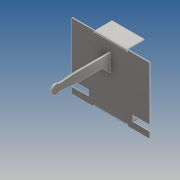
# Autodesk Inventor part: Porta actuador
Saved by Autodesk Inventor 2016 (Build 200138000, 138)
## iProperties
Created: 2016-05-25
Part Number: Porta actuador
Material: Stainless Steel
Document SubType Name: Sheet Metal
Designer: Familia
Density: 8 g/cm^3
Sheet Metal Rule: Default_mm
Appearance: Semi-Polished
Author: Familia
Autodesk Inventor part; units mm, degrees
note: some values were not read from the file. Chosen so that the rebuilt part matches the saved one: relief shape of "Plate2"; relief shape of "Plate3".
ref_plane "YZ Plane" through (0, 0, 0) normal (1, 0, 0) x (0, 1, 0)
ref_plane "XZ Plane" through (0, 0, 0) normal (0, 1, 0) x (-1, 0, 0)
ref_plane "XY Plane" through (0, 0, 0) normal (0, 0, 1) x (1, 0, 0)
sketch "Sketch1" plane through (0, 0, 0) normal (0, 1, 0) x (-1, 0, 0)
  line L0 (26.5, -22.5) -> (-26.5, -22.5)
  line L1 (-26.5, -22.5) -> (-26.5, 22.5)
  line L2 (-26.5, 22.5) -> (26.5, 22.5)
  line L3 (26.5, 22.5) -> (26.5, -22.5)
  line L4 (26.5, -22.5) -> (-26.5, 22.5) construction
  line L5 (-26.5, -22.5) -> (26.5, 22.5) construction
  line L6 (-23.1815, -2.0327) -> (-17.2605, -2.0327)
  line L7 (-17.2605, -2.0327) -> (-17.2605, -20.329)
  line L8 (-17.2605, -20.329) -> (-23.1815, -20.329)
  line L9 (-23.1815, -20.329) -> (-23.1815, -2.0327)
  line L10 (15.4694, -2.0327) -> (21.0827, -2.0327)
  line L11 (21.0827, -2.0327) -> (21.0827, -20.329)
  line L12 (21.0827, -20.329) -> (15.4694, -20.329)
  line L13 (15.4694, -20.329) -> (15.4694, -2.0327)
  line L14 (1, 11) -> (0, 11)
  line L15 (0, 11) -> (0, 3)
  line L16 (0, 3) -> (1, 3)
  line L17 (1, 3) -> (1, 11)
  point P0 (0, 0)
  point P1 (0, 0)
  dimension "d0" = 53
  dimension "d1" = 45
  dimension "d43" = 8
  dimension "d44" = 1
  dimension "d45" = 3
  measures "d0" distance of L1.end L2.end
  measures "d1" distance of L2.end L0.start
  measures "d43" distance of L16.end L14.start
  measures "d44" distance of L14.start L14.end
  measures "d45" distance of point (0, 0) L15.end
extrude "Plate1" add sketch "Sketch1" along normal blind 0.5 contours L0 L1 L2 L3 | L6 L7 L8 L9 | L10 L11 L12 L13 | L17 L16 L15 L14
sketch "Sketch2" plane through (26.5, 0, 22) normal (0, 0, 1) x (1, 0, 0)
  line L0 (-37.5, 0) -> (-15.5, 0)
  line L1 (-15.5, 0) -> (-15.5, 12)
  line L2 (-15.5, 12) -> (-37.5, 12)
  line L3 (-37.5, 12) -> (-37.5, 0)
  constraints: 8 end point
edge flange "Flange1" height 12 angle 90 thickness 0.5 bend radius 0.5 thickness toward (0, 0, 1) relief straight relief width 0.5 relief depth 0.25 edges at (0, 0.5, 22.5) wall of the first edge with corners at (-11, 0, 22) (11, 0, 22) (11, 12, 22) (-11, 12, 22)
bend "Bend1"
corner "Corner1"
sketch "Sketch3" plane through (26.5, 0, -22) normal (0, 0, -1) x (-1, 0, 0)
  line L0 (37.5, 0) -> (15.5, 0)
  line L1 (15.5, 0) -> (15.5, -12)
  line L2 (15.5, -12) -> (37.5, -12)
  line L3 (37.5, -12) -> (37.5, 0)
  constraints: 8 end point
edge flange "Flange2" height 12 angle 90 thickness 0.5 bend radius 0.5 thickness toward (0, 0, -1) relief straight relief width 0.5 relief depth 0.25 edges at (0, 0, -22.5) wall of the first edge with corners at (-11, 0, -22) (11, 0, -22) (11, 12, -22) (-11, 12, -22)
bend "Bend2"
corner "Corner2"
sketch "Sketch4" plane through (0, 0, 0) normal (0, -1, 0) x (1, 0, 0)
  line L0 (-32.114, -14.2) -> (-15, -14.2)
  line L1 (-15, -14.2) -> (-15, -18.2)
  line L2 (-15, -18.2) -> (-32.114, -18.2)
  line L3 (-32.114, -18.2) -> (-32.114, -14.2)
  line L4 (15, -14.2) -> (31.1601, -14.2)
  line L5 (31.1601, -14.2) -> (31.1601, -18.2)
  line L6 (31.1601, -18.2) -> (15, -18.2)
  line L7 (15, -18.2) -> (15, -14.2)
  line L8 (26.5, -22.5) -> (26.5, 22.5) projected
  line L9 (-26.5, 22.5) -> (-26.5, -22.5) projected
  line L10 (-15, -16.2) -> (0, -16.2) construction
  line L11 (0, -16.2) -> (15, -16.2) construction
  line L12 (0, 0) -> (0, -16.2) construction
  dimension "d25" = 4.3
  dimension "d26" = 4.3
  dimension "d27" = 30
  dimension "d29" = 4
  constraints: 22 end point, 4 parallel, 3 horizontal, 2 midpoint, 2 perpendicular, 1 collinear, 1 point on line, 1 vertical
  measures "d25" vertical distance of L2.end L9.end
  measures "d26" distance from line of L6 L8.start
  measures "d27" distance between parallel lines of L7 L1
  measures "d29" distance of L4.end L5.end
extrude "Cut1" cut sketch "Sketch4" against normal blind 0.5
sketch "Sketch5" plane through (0, 0.5, 0) normal (0, 1, 0) x (1, 0, 0)
  line L0 (21.5, 1.2) -> (15.5, 1.2)
  line L1 (15.5, 1.2) -> (15.5, 11.2)
  line L2 (15.5, 11.2) -> (21.5, 11.2)
  line L3 (21.5, 11.2) -> (21.5, 1.2)
  line L4 (0, 0) -> (0, 26.5728) construction
  line L5 (26.5, 14.2) -> (26.5, -22.5) projected
  line L6 (26.5, 14.2) -> (15, 14.2) projected
  line L7 (-21.5, 1.2) -> (-15.5, 1.2)
  line L8 (-15.5, 1.2) -> (-15.5, 11.2)
  line L9 (-15.5, 11.2) -> (-21.5, 11.2)
  line L10 (-21.5, 11.2) -> (-21.5, 1.2)
  dimension "d37" = 5
  dimension "d38" = 6
  dimension "d39" = 3
  dimension "d40" = 10
  constraints: 18 end point, 4 symmetric about line, 2 parallel, 1 horizontal, 1 perpendicular, 1 vertical
  measures "d37" distance between parallel lines of L3 L5
  measures "d38" distance of L0.start L0.end
  measures "d39" distance between parallel lines of L6 L2
  measures "d40" distance between parallel lines of L2 L0
extrude "Extrusion1" add sketch "Sketch5" along normal blind 5
sketch "Sketch6" plane through (15.5, 0.5, -1.2) normal (0, 0, 1) x (1, 0, 0)
  circle A0 centre (3, 2.5) radius 1.5
  line L0 (6, 0) -> (6, 5) projected
  line L1 (0, 5) -> (6, 5) projected
  line L2 (0, 0) -> (0, 5) projected
  line L3 (6, 2.5) -> (3, 2.5) construction
  line L4 (3, 2.5) -> (0, 2.5) construction
  line L5 (-15.5, -0.5) -> (-15.5, 16.3253) construction
  circle A1 centre (-34, 2.5) radius 1.5
  dimension "d34" = 3
  constraints: 6 end point, 2 centre point, 2 horizontal, 2 midpoint, 1 collinear, 1 symmetric about line, 1 vertical, 1 other
  measures "d34" diameter of A0
extrude "Extrusion2" cut sketch "Sketch6" against normal through all
fillet "Fillet1" radius 3 4 edges at (21.5, 5.5, -6.2) (15.5, 5.5, -6.2) (-15.5, 5.5, -6.2) (-21.5, 5.5, -6.2)
sketch "Sketch7" plane through (0, 0, 0) normal (0, -1, 0) x (1, 0, 0)
  line L0 (-1, 15) -> (0, 15)
  line L1 (0, 15) -> (0, 3)
  line L2 (0, 3) -> (-1, 3)
  line L3 (-1, 3) -> (-1, 15)
  point P0 (0, 0)
  dimension "d46" = 1
  dimension "d47" = 12
  dimension "d48" = 3
  constraints: 8 end point, 2 parallel, 1 horizontal, 1 perpendicular, 1 vertical alignment
  measures "d46" distance of L0.start L0.end
  measures "d47" distance of L2.end L0.start
  measures "d48" distance from line of point (0, 0) L2
extrude "Extrusion3" add sketch "Sketch7" along normal blind 40
sketch "Sketch8" plane through (0, 0, 15) normal (1, 0, 0) x (0, 0, -1)
  arc A0 (0.9, -34.6455) -> (5.4, -34.6455) centre (3.15, -36.85) ccw
  line L0 (12, -40) -> (0, -40) projected
  line L1 (0, 0) -> (0, -40) construction
  line L2 (0.9, -34.6455) -> (0, -24.6455)
  line L3 (5.4, -34.6455) -> (6.35, -24.0899)
  line L4 (3.15, -36.85) -> (3.15, 3.4325) construction
  line L5 (6.35, -24.0899) -> (6.35, -6)
  line L6 (6.35, -6) -> (12, 0)
  line L7 (12, 0) -> (0, 0)
  line L8 (0, 0) -> (0, -24.6455)
  line L9 (12, 0) -> (12, -40) construction
  line L10 (12, 0) -> (12, -48.2651)
  line L11 (12, -48.2651) -> (-5.7292, -48.2651)
  line L12 (-5.7292, -48.2651) -> (-5.7292, -24.6455)
  line L13 (-5.7292, -24.6455) -> (0, -24.6455)
  point P0 (15, 0)
  dimension "d51" = 6.3
  dimension "d52" = 4.5
  dimension "d53" = 10
  dimension "d54" = 6.35
  dimension "d55" = 6
  constraints: 22 end point, 4 perpendicular, 3 vertical, 2 point on circle, 2 tangent, 1 centre point, 1 collinear, 1 horizontal alignment, 1 point on line, 1 other
  measures "d51" diameter of A0
  measures "d52" distance of L3.start L2.start
  measures "d53" vertical distance of L2.start L2.end
  measures "d54" distance between parallel lines of L5 L1
  measures "d55" vertical distance of L6.end L5.end
extrude "Extrusion4" cut sketch "Sketch8" against normal through all contours A0 L0 L10 L11 L12 L13 L2 | A0 L3 L5 L6 L10 L0
equation "\"d30\" = Thickness"
equation "\"d3\" = BendReliefWidth"
equation "\"d4\" = BendReliefDepth"
equation "\"d5\" = MinimumRemnant"
equation "\"d6\" = BendRadius"
equation "\"d10\" = BendRadius"
equation "\"d11\" = CornerReliefSize"
equation "\"d12\" = GapSize"
equation "\"d13\" = JacobiRadiusSize"
equation "\"d14\" = BendReliefWidth"
equation "\"d15\" = BendReliefDepth"
equation "\"d16\" = MinimumRemnant"
equation "\"d17\" = BendRadius"
equation "\"d21\" = BendRadius"
equation "\"d22\" = CornerReliefSize"
equation "\"d23\" = GapSize"
equation "\"d24\" = JacobiRadiusSize"
equation "\"BendRadius\" = Thickness"
equation "\"BendReliefWidth\" = Thickness"
equation "\"BendReliefDepth\" = 0.5 * Thickness"
equation "\"CornerReliefSize\" = 4 * Thickness"
equation "\"MinimumRemnant\" = 2 * Thickness"
equation "\"TransitionRadius\" = BendRadius"
equation "\"JacobiRadiusSize\" = BendRadius"
equation "\"GapSize\" = Thickness"
equation "\"d2\" = BendRadius"
equation "\"Thickness\" = 0.5"
body "Solid1"
